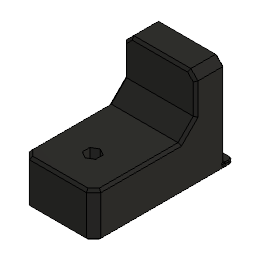
y_idler_bracket (Autodesk Fusion 360 design; units mm, degrees)
Autodesk Fusion 360 part; units mm, degrees
note: some values were not read from the file. Chosen so that the rebuilt part matches the saved one: which face or edge a step refers to; a direction; which pieces of a blend or face edit are solid. Set by a fixed rule: which sketch regions a step uses.
sketch "Sketch1" plane through (0, 0, 0) normal (0, 0, 1) x (1, 0, 0)
  line L0 (0, 13) -> (0, -13) construction
  circle A0 centre (0, 13) radius 1.7
  circle A1 centre (0, -13) radius 1.7
  line L1 (-15, 14.35) -> (15, 14.35)
  line L2 (15, 14.35) -> (15, -21.5)
  line L3 (15, -21.5) -> (-15, -21.5)
  line L4 (-15, -21.5) -> (-15, 14.35)
  line L5 (-15, 19.35) -> (15, 19.35)
  line L6 (15, 19.35) -> (15, 14.35)
  line L7 (-15, 14.35) -> (-15, 19.35)
  line L8 (-15, -18.5) -> (-12, -21.5)
  line L9 (15, -18.5) -> (12, -21.5)
  line L10 (15, 17) -> (-15, 17)
  line L11 (-0.7632, 11.3) -> (0.7632, 11.3)
  line L12 (-1.2042, 11.8) -> (1.2042, 11.8)
  line L13 (1.2704, 11.8704) -> (0.7632, 11.3)
  line L14 (-1.2704, 11.8704) -> (-0.7632, 11.3)
  line L15 (-0.7042, -14.7) -> (0.7042, -14.7)
  line L16 (1.2021, -14.2021) -> (0.7042, -14.7)
  line L17 (0, -13) -> (1.2021, -14.2021) construction
  line L18 (0, -13) -> (-1.2021, -14.2021) construction
  line L19 (-1.2021, -14.2021) -> (-0.7042, -14.7)
  circle A2 centre (0, -13) radius 2.25
  line L20 (-1.591, -14.591) -> (-0.932, -15.25)
  line L21 (1.591, -14.591) -> (0.932, -15.25)
  line L22 (0.932, -15.25) -> (-0.932, -15.25)
  line L23 (-1.4142, -14.75) -> (1.4142, -14.75)
  line L24 (-1.2042, -14.2) -> (1.2042, -14.2) construction
  circle A3 centre (0, 13) radius 2.25
  line L25 (1.0102, 10.75) -> (-1.0102, 10.75)
  line L26 (-1.6814, 11.5049) -> (-1.0102, 10.75)
  line L27 (1.6814, 11.5049) -> (1.0102, 10.75)
  point P0 (0, -13)
  point P1 (0, 13)
  point P2 (0, -15.25)
  point P3 (0, 10.75)
  dimension "d1" = 26
  dimension "d2" = 3.4
  dimension "d3" = 3.4
  dimension "d4" = 30
  dimension "d6" = 8.5
  dimension "d7" = 15
  dimension "d8" = 5
  dimension "d10" = 45
  dimension "d11" = 3
  dimension "d38" = 40.85
  dimension "d60" = 2.35
  dimension "d74" = 0.5
  dimension "d81" = 4.5
  dimension "d82" = 0.5
  dimension "d83" = 0.5
  dimension "d84" = 135
  dimension "d90" = 4.5
  constraint vertical L0
  constraint coincident L0.start A0.centre
  constraint midpoint origin L0
  constraint coincident P0 L0.end
  constraint horizontal L1
  constraint vertical L2
  constraint horizontal L3
  constraint vertical L4
  constraint horizontal L5
  constraint vertical L6
  constraint vertical L7
  constraint coincident L1.start L4.end
  constraint coincident L1.end L2.start
  constraint coincident L4 L8.start
  constraint coincident L3 L8.end
  constraint symmetric L0 L8.start L9.start
  constraint symmetric L0 L8.end L9.end
  constraint coincident P1 L0.start
  constraint coincident L6 L10.start
  constraint coincident L7 L10.end
  constraint horizontal L10
  constraint horizontal L11
  constraint tangent A0 L11
  constraint coincident A0 L12.start
  constraint coincident A0 L12.end
  constraint horizontal L12
  constraint coincident A0 L13.start
  constraint tangent A0 L13
  constraint coincident L11.end L13.end
  constraint coincident A0 L14.start
  constraint tangent A0 L14
  constraint coincident L11.start L14.end
  constraint horizontal L15
  constraint tangent A1 L15
  constraint coincident A1 L16.start
  constraint tangent A1 L16
  constraint coincident L15.end L16.end
  constraint perpendicular L16 L17
  constraint coincident L16.start L17.end
  constraint perpendicular L17 L18
  constraint coincident A1 L18.end
  constraint tangent A1 L19
  constraint coincident L15.start L19.end
  constraint perpendicular L18 L19
  constraint coincident A2 L20.start
  constraint tangent A2 L20
  constraint coincident A2 L21.start
  constraint tangent A2 L21
  constraint horizontal L22
  constraint coincident L20.end L22.end
  constraint tangent A2 L22
  constraint coincident A2 L23.start
  constraint coincident A2 L23.end
  constraint horizontal L23
  constraint coincident A1 L24.start
  constraint coincident A1 L24.end
  constraint horizontal L24
  constraint coincident A2 P2
  constraint coincident L0 P2
  constraint midpoint L22 P2
  constraint parallel L19 L20
  constraint concentric A0 A3
  constraint horizontal L25
  constraint coincident A3 P3
  constraint coincident L0 P3
  constraint midpoint L25 P3
  constraint coincident A3 L26.start
  constraint tangent A3 L26
  constraint coincident A3 L27.start
  constraint tangent A3 L27
  constraint coincident L25.start L27.end
  constraint coincident L25.end L26.end
  constraint parallel L14 L26
  constraint parallel L13 L27
  measures "d1" distance of L0.start P0
  measures "d2" diameter of A0
  measures "d3" diameter of A1
  measures "d4" distance of L1.start L1.end
  measures "d6" distance of P0 L3
  measures "d7" distance of P0 L2
  measures "d8" distance of L5.end L1.end
  measures "d10" angle of L3 L8
  measures "d11" distance of L3.end L8.end
  measures "d38" distance of L3.end L5.start
  measures "d60" distance of L5.end L10.start
  measures "d74" distance of L11 L12
  measures "d81" diameter of A2
  measures "d82" distance of L22 L23
  measures "d83" distance of L15 L24
  measures "d84" angle of L0 L17
  measures "d90" diameter of A3
extrude "Extrude1" add sketch "Sketch1" along normal blind 11.8 contours A0 L1 L12 | A0 L1 L11 L13 L14 A3 | A0 L11 L14 | A0 L12 | A0 L1 A3 | A0 L1 | A0 L11 L13 | L1 L2 L3 L4 L8 L9 A3 L25 L26 L27 | L1 L6 L7 L10 A3 | A3 L25 L26 | L5 L6 L7 L10 | A3 L25 L27 | A1 | A1 L15 L19 | A1 L15 L16 | A2 L23 | A2 L20 L22 | A2 L21 L22 | A2 L23
extrude "Extrude2" add sketch "Sketch1" along normal blind 54.6 contours A0 L1 A3 | A0 L1 | L1 L6 L7 L10 A3 | L5 L6 L7 L10
sketch "Sketch2" plane through (0, 14.35, 0) normal (0, -1, 0) x (1, 0, 0)
  line L0 (-15, 11.8) -> (15, 11.8)
  line L1 (15, 11.8) -> (15, 54.6)
  line L2 (15, 54.6) -> (-15, 54.6)
  line L3 (-15, 54.6) -> (-15, 11.8)
  circle A0 centre (0, 40) radius 1.6
  circle A1 centre (0, 40) radius 2.25
  dimension "d16" = 30
  dimension "d17" = 42.8
  dimension "d18" = 3.2
  dimension "d19" = 15
  dimension "d20" = 14.6
  dimension "d76" = 4.5
  constraint concentric A0 A1
  measures "d16" distance of L1.end L2.end
  measures "d17" distance of L0.end L1.end
  measures "d18" diameter of A0
  measures "d19" horizontal distance of L1.end A0.centre
  measures "d20" vertical distance of L1.end A0.centre
  measures "d76" diameter of A1
extrude "Extrude3" cut sketch "Sketch2" against normal blind 13 contours A0
extrude "Extrude6" cut sketch "Sketch1" along normal blind 6.8 contours A0 L1 L12 | A0 L11 L14 | A0 L12 | A0 L1 | A0 L11 L13 | A1 | A1 L15 L19 | A1 L15 L16
extrude "Extrude9" add sketch "Sketch1" against normal blind 4.2 contours L5 L6 L7 L10
extrude "Extrude11" cut sketch "Sketch2" against normal blind 5 contours A0 | A1
chamfer "Chamfer16" distance 0.625 angle 45 1 edges at (-2.0977, 19.35, 39.1864)
sketch "Sketch5" plane through (-15, 0, 0) normal (-1, 0, 0) x (0, -1, 0)
  line L0 (-17, 0) -> (18.5, 0)
  line L1 (18.5, 0) -> (18.5, 11.8)
  line L2 (18.5, 11.8) -> (-14.35, 11.8)
  line L3 (-14.35, 11.8) -> (-14.35, 54.6)
  line L4 (-14.35, 54.6) -> (-19.35, 54.6)
  line L5 (-19.35, 54.6) -> (-19.35, -4.2)
  line L6 (-19.35, -4.2) -> (-17, -4.2)
  line L7 (-17, -4.2) -> (-17, 0)
  circle A0 centre (-17, 0) radius 0.5
  dimension "d63" = 1
  constraint coincident L0.start L7.end
  measures "d63" diameter of A0
extrude "Extrude10" cut sketch "Sketch5" against normal blind 30 contours L0 L7 A0 | L0 L7 A0
chamfer "Chamfer1" distance 3 angle 45 2 edges at (15, 16.85, 54.6) (-15, 16.85, 54.6)
chamfer "Chamfer11" distance 20 angle 45 1 edges at (0, 14.35, 11.8)
chamfer "Chamfer2" distance 1 angle 45 12 edges at (-15, 14.35, 41.7) (-13.5, 14.35, 53.1) (0, 14.35, 54.6) (13.5, 14.35, 53.1) (15, 14.35, 41.7) (15, -12.075, 11.8) (13.5, -20, 11.8) (0, -21.5, 11.8) (-13.5, -20, 11.8) (-15, -12.075, 11.8) (-15, 4.35, 21.8) (15, 4.35, 21.8)
fillet "Fillet2" radius 2 2 edges at (-15, 18.175, -4.2) (15, 18.175, -4.2)
fillet "Fillet3" radius 0.5 2 edges at (0, 17, -0.5) (0, 16.5, 0)
chamfer "Chamfer14" distance 0.4 angle 45 16 edges at (15, -1.183, 0) (15, 16.384, 0.067) (15, 17.3536, 0.3536) (15, 17.067, -0.616) (15, 17, -1.533) (14.4142, 17, -3.6142) (0, 17, -4.2) (-14.4142, 17, -3.6142) (-15, 17, -1.533) (-15, 17.067, -0.616) (-15, 17.3536, 0.3536) (-15, 16.384, 0.067) (-15, -1.183, 0) (13.5, -20, 0) (0, -21.5, 0) (-13.5, -20, 0)
chamfer "Chamfer15" distance 1 angle 45 8 edges at (-15, 19.35, 24.7) (-14.4142, 19.35, -3.6142) (0, 19.35, -4.2) (14.4142, 19.35, -3.6142) (15, 19.35, 24.7) (-13.5, 19.35, 53.1) (0, 19.35, 54.6) (13.5, 19.35, 53.1)
chamfer "Chamfer17" distance 0.4 angle 45 1 edges at (-2.0977, 14.35, 40.8136)
extrude "Extrude13" cut sketch "Sketch1" along normal blind 5 contours A0 L1 L11 L13 L14 A3 | A0 L11 L14 | A0 L12 | A0 L1 A3 | A0 L11 L13 | A3 L25 L26 | A3 L25 L27 | A1 | A1 L15 L19 | A1 L15 L16 | A2 L23 | A2 L20 L22 | A2 L21 L22 | A2 L23
chamfer "Chamfer20" distance 0.525 angle 45 8 edges at (1.0168, 11.5852, 5) (0, 14.7, 5) (-1.0168, 11.5852, 5) (0, 11.3, 5) (0, -11.3, 5) (0.9531, -14.451, 5) (-0.9531, -14.451, 5) (0, -14.7, 5)
chamfer "Chamfer21" distance 0.4 angle 45 6 edges at (1.3458, 11.1274, 0) (0, 15.25, 0) (-1.3458, 11.1274, 0) (0, -10.75, 0) (-1.2615, -14.9205, 0) (1.2615, -14.9205, 0)
move_body "Move1" bodies 1 to x (-1, 0, 0) y (0, 0, -1) z (0, -1, 0) at (-30, -21.5, -21.5)
move_body "Move2" bodies 1 to x (1, 0, 0) y (0, 1, 0) z (0, 0, 1) at (30, 46.7, 40.85)
delete_face "DeleteFace1" 1 faces at (14.6667, -13.0619, 4.3333)
delete_face "DeleteFace2" 1 faces at (13.8619, -26.5953, 4.6667)
delete_face "DeleteFace3" 1 faces at (4.4714, -28.7333, 4.6667)
delete_face "DeleteFace4" 1 faces at (-12.1953, -28.2619, 4.6667)
delete_face "DeleteFace5" 1 faces at (14.3333, 0.5381, 11.6667)
delete_face "DeleteFace6" 1 faces at (-14.3333, 0.5381, 11.6667)
delete_face "DeleteFace7" 1 faces at (-14.3333, -13.8667, 4.6667)
extrude "Extrude14" add 1 faces at (-0.066, -25.4142, 5) along direction (0, 0, 1) blind 10
delete_face "DeleteFace8" 1 faces at (-1.9548, -16.6138, 0.2083)
sketch "Sketch6" plane through (0, 0, 0) normal (0, 0, -1) x (1, 0, 0)
  line L0 (11.5858, 28.4) -> (-11.5858, 28.4)
  line L1 (-11.5858, 28.4) -> (-14, 25.9858)
  line L2 (-14, 25.9858) -> (-14, -27.4)
  arc A0 (-14, -27.4) -> (-13, -28.4) centre (-13, -27.4) ccw
  line L3 (-13, -28.4) -> (13, -28.4)
  arc A1 (13, -28.4) -> (14, -27.4) centre (13, -27.4) ccw
  line L4 (14, -27.4) -> (14, 25.9858)
  line L5 (14, 25.9858) -> (11.5858, 28.4)
  circle A2 centre (0, 14.8) radius 2.25
  circle A3 centre (0, 14.8) radius 3.5
  circle A4 centre (0, 14.8) radius 1.6
  dimension "d98" = 7
  dimension "d99" = 3.2
  constraint concentric A2 A3
  constraint concentric A3 A4
  measures "d98" diameter of A3
  measures "d99" diameter of A4
extrude "Extrude15" add sketch "Sketch6" against normal up to surface (15 mm away) contours A2 | A3
extrude "Extrude16" add 1 faces at (-0.0399, -25.0652, 15) along direction (0, 0, 1) blind 3.6
sketch "Sketch7" plane through (15, 0, 0) normal (1, 0, 0) x (0, 1, 0)
  line L0 (14.4, 26) -> (-6.6, 5)
  line L1 (-6.6, 5) -> (-6.6, 18.6)
  line L2 (-6.6, 18.6) -> (-26.4, 18.6)
  line L3 (-26.4, 18.6) -> (-26.4, 1)
  line L4 (-26.4, 1) -> (27.4, 1)
  line L5 (27.4, 1) -> (27.4, 1.95)
  line L6 (27.4, 1.95) -> (26.066, 1.95)
  arc A0 (26.066, 1.95) -> (25.9794, 1.9) centre (26.066, 1.85) ccw
  arc A1 (24.75, 3.1294) -> (25.9794, 1.9) centre (25.2, 2.35) ccw
  arc A2 (24.75, 3.1294) -> (24.8, 3.216) centre (24.7, 3.216) ccw
  line L7 (24.8, 3.216) -> (24.8, 37.85)
  line L8 (24.8, 37.85) -> (14.4, 37.85)
  line L9 (14.4, 37.85) -> (14.4, 26)
  line L10 (-6.6, 18.6) -> (7, 18.6)
  constraint coincident L1.end L2.start
  constraint coincident L0 L10.end
  constraint perpendicular L1 L10
extrude "Extrude17" add sketch "Sketch7" against normal up to surface (30 mm away) contours L0 L1 L10
sketch "Sketch8" plane through (0, 0, 18.6) normal (0, 0, 1) x (-1, 0, 0)
  circle A0 centre (0, 14.8) radius 1.6
  line L0 (15, 26.4) -> (12, 29.4)
  line L1 (12, 29.4) -> (-12, 29.4)
  line L2 (-12, 29.4) -> (-15, 26.4)
  line L3 (-15, 26.4) -> (-15, -7)
  line L4 (-15, -7) -> (15, -7)
  line L5 (15, -7) -> (15, 26.4)
  circle A1 centre (0, 14.8) radius 1.55
  line L6 (2.75, 16.3877) -> (0, 17.9754)
  line L7 (0, 17.9754) -> (-2.75, 16.3877)
  line L8 (-2.75, 16.3877) -> (-2.75, 13.2123)
  line L9 (-2.75, 13.2123) -> (0, 11.6246)
  line L10 (0, 11.6246) -> (2.75, 13.2123)
  line L11 (2.75, 13.2123) -> (2.75, 16.3877)
  circle A2 centre (0, 14.8) radius 1.6
  line L12 (15, 26.4) -> (12, 29.4)
  line L13 (12, 29.4) -> (-12, 29.4)
  line L14 (-12, 29.4) -> (-15, 26.4)
  line L15 (-15, 26.4) -> (-15, -7)
  line L16 (-15, -7) -> (15, -7)
  line L17 (15, -7) -> (15, 26.4)
  point P0 (0, 14.8)
  dimension "d107" = 2.75
  constraint coincident P0 A0.centre
  measures "d107" distance of P0 L11
extrude "Extrude18" cut sketch "Sketch8" against normal blind 5 contours L6 L7 L8 L9 L10 L11
chamfer "Chamfer23" distance 1 angle 45 7 edges at (15, 10.7, 22.3) (15, -9.7, 18.6) (13.5, -27.9, 18.6) (0, -29.4, 18.6) (-13.5, -27.9, 18.6) (-15, -9.7, 18.6) (-15, 10.7, 22.3)
sketch "Sketch10" plane through (0, 0, 0) normal (0, 0, -1) x (1, 0, 0)
  circle A0 centre (0, 14.8) radius 1.6
  line L0 (11.5858, 28.4) -> (-11.5858, 28.4)
  line L1 (-11.5858, 28.4) -> (-14, 25.9858)
  line L2 (-14, 25.9858) -> (-14, -27.4)
  arc A1 (-14, -27.4) -> (-13, -28.4) centre (-13, -27.4) ccw
  line L3 (-13, -28.4) -> (13, -28.4)
  arc A2 (13, -28.4) -> (14, -27.4) centre (13, -27.4) ccw
  line L4 (14, -27.4) -> (14, 25.9858)
  line L5 (14, 25.9858) -> (11.5858, 28.4)
  circle A3 centre (0, 14.8) radius 3.1
  dimension "d117" = 6.2
  constraint concentric A0 A3
  measures "d117" diameter of A3
extrude "Extrude20" cut sketch "Sketch10" against normal blind 3 contours A3
chamfer "Chamfer27" distance 0.2 angle 45 1 edges at (-2.8902, -15.921, 0)
chamfer "Chamfer28" distance 0.2 angle 45 1 edges at (-1.4917, -14.2214, 3)
sketch "Sketch11" plane through (0, 0, 3) normal (0, 0, -1) x (1, 0, 0)
  circle A0 centre (0, 14.8) radius 3.1
  circle A1 centre (0, 14.8) radius 1.8 construction
  line L0 (0, 14.8) -> (1, 14.8) construction
  line L1 (-2.5232, 12.999) -> (2.5232, 12.999)
  line L2 (-2.5232, 16.601) -> (2.5232, 16.601)
  line L3 (0, 14.8) -> (0, 12.999) construction
  line L4 (0, 14.8) -> (0, 16.601) construction
  dimension "d122" = 1.801
  dimension "d123" = 1.801
  constraint coincident A0.centre A1.centre
  constraint parallel L0 L1
  constraint parallel L0 L2
  constraint perpendicular L1 L3
  constraint coincident L1 L3.end
  constraint perpendicular L2 L4
  constraint coincident L2 L4.end
  constraint coincident A0 L1.start
  constraint coincident A0 L1.end
  constraint coincident A0 L2.start
  constraint coincident A0 L2.end
  measures "d122" distance of A0.centre L3.end
  measures "d123" distance of A0.centre L4.end
extrude "Extrude21" cut sketch "Sketch11" against normal blind 0.2 contours A0 L1 L2
sketch "Sketch12" plane through (0, 0, 3.2) normal (0, 0, -1) x (1, 0, 0)
  circle A0 centre (0, 14.8) radius 1.6 construction
  line L0 (-2.5232, 12.999) -> (2.5232, 12.999)
  arc A1 (2.5232, 12.999) -> (2.5232, 16.601) centre (0, 14.8) ccw
  line L1 (2.5232, 16.601) -> (-2.5232, 16.601)
  arc A2 (-2.5232, 16.601) -> (-2.5232, 12.999) centre (0, 14.8) ccw
  line L2 (0, 14.8) -> (1, 14.8) construction
  line L3 (0, 14.8) -> (0, 15.8) construction
  line L4 (1.601, 12.999) -> (1.601, 16.601)
  line L5 (-1.601, 12.999) -> (-1.601, 16.601)
  line L6 (0, 14.8) -> (1.601, 14.8) construction
  line L7 (0, 14.8) -> (-1.601, 14.8) construction
  dimension "d126" = 90
  dimension "d127" = 1.601
  dimension "d128" = 1.601
  constraint coincident A0.centre A1.centre
  constraint parallel L3 L4
  constraint parallel L3 L5
  constraint perpendicular L4 L6
  constraint coincident L4 L6.end
  constraint perpendicular L5 L7
  constraint coincident L5 L7.end
  constraint coincident L0 L4.start
  constraint coincident L1 L4.end
  constraint coincident L0 L5.start
  constraint coincident L1 L5.end
  measures "d126" angle of L2 L3
  measures "d127" distance of A0.centre L6.end
  measures "d128" distance of A0.centre L7.end
extrude "Extrude22" cut sketch "Sketch12" against normal blind 0.2 contours L0 L1 L4 L5
extrude "Extrude23" add 1 faces at (-1.2572, -13.4199, 3.4) along direction (0, 0, -1) up to surface (0.2 mm away)
extrude "Extrude24" add 3 faces at (2.1007, -14.8, 3.2) (-2.0982, -14.7289, 3.2) (-1.2572, -13.4199, 3.2) along direction (0, 0, -1) up to surface end surface through (0, 0, 3) normal (0, 0, -1) offset 0
delete_face "DeleteFace17" 1 faces at (3.2173, -14.4781, 0.0667)
sketch "Sketch13" plane through (0, 0, 0) normal (0, 0, -1) x (1, 0, 0)
  line L0 (11.5858, 28.4) -> (-11.5858, 28.4)
  line L1 (-11.5858, 28.4) -> (-14, 25.9858)
  line L2 (-14, 25.9858) -> (-14, -27.4)
  arc A0 (-14, -27.4) -> (-13, -28.4) centre (-13, -27.4) ccw
  line L3 (-13, -28.4) -> (13, -28.4)
  arc A1 (13, -28.4) -> (14, -27.4) centre (13, -27.4) ccw
  line L4 (14, -27.4) -> (14, 25.9858)
  line L5 (14, 25.9858) -> (11.5858, 28.4)
  circle A2 centre (0, 14.8) radius 3.1
  line L6 (-2.75, 13.2123) -> (0, 11.6246)
  line L7 (0, 11.6246) -> (2.75, 13.2123)
  line L8 (2.75, 13.2123) -> (2.75, 16.3877)
  line L9 (2.75, 16.3877) -> (0, 17.9754)
  line L10 (0, 17.9754) -> (-2.75, 16.3877)
  line L11 (-2.75, 16.3877) -> (-2.75, 13.2123)
  point P0 (0, 14.8)
  dimension "d135" = 2.75
  constraint coincident P0 A2.centre
  measures "d135" distance of P0 L11
move_face "OffsetFaces1" offset 1.3 1 faces at (3.0846, -14.4913, 1)
extrude "Extrude25" cut sketch "Sketch13" against normal blind 2.4 contours A2 L6 L7 L8 L9 L10 L11
chamfer "Chamfer29" distance 0.4 angle 45 12 edges at (1.375, -12.4184, 0) (0, -11.7, 0) (-1.375, -12.4184, 0) (-2.6847, -13.25, 0) (-2.75, -14.8, 0) (-2.6847, -16.35, 0) (-1.375, -17.1816, 0) (0, -17.9, 0) (1.375, -17.1816, 0) (2.6847, -16.35, 0) (2.75, -14.8, 0) (2.6847, -13.25, 0)
extrude "Extrude26" add 1 faces at (1.1833, -16.8496, 13.6) along direction (0, 0, 1) blind 1
sketch "Sketch14" plane through (0, 0, 2.4) normal (0, 0, -1) x (1, 0, 0)
  circle A0 centre (0, 14.8) radius 1.8 construction
  arc A1 (-2.6142, 16.4661) -> (-2.75, 16.2309) centre (0, 14.8) ccw
  line L0 (-2.75, 16.2309) -> (-2.75, 13.3691)
  arc A2 (-2.75, 13.3691) -> (-2.6142, 13.1339) centre (0, 14.8) ccw
  line L1 (-2.6142, 13.1339) -> (-0.1358, 11.703)
  arc A3 (-0.1358, 11.703) -> (0.1358, 11.703) centre (0, 14.8) ccw
  line L2 (0.1358, 11.703) -> (2.6142, 13.1339)
  arc A4 (2.6142, 13.1339) -> (2.75, 13.3691) centre (0, 14.8) ccw
  line L3 (2.75, 13.3691) -> (2.75, 16.2309)
  arc A5 (2.75, 16.2309) -> (2.6142, 16.4661) centre (0, 14.8) ccw
  line L4 (2.6142, 16.4661) -> (0.1358, 17.897)
  arc A6 (0.1358, 17.897) -> (-0.1358, 17.897) centre (0, 14.8) ccw
  line L5 (-0.1358, 17.897) -> (-2.6142, 16.4661)
  line L6 (0, 14.8) -> (1, 14.8) construction
  line L7 (-2.3806, 12.999) -> (2.3806, 12.999)
  line L8 (-2.3806, 16.601) -> (2.3806, 16.601)
  line L9 (0, 14.8) -> (0, 12.999) construction
  line L10 (0, 14.8) -> (0, 16.601) construction
  dimension "d142" = 1.801
  dimension "d143" = 1.801
  constraint coincident A0.centre A1.centre
  constraint parallel L6 L7
  constraint parallel L6 L8
  constraint perpendicular L7 L9
  constraint coincident L7 L9.end
  constraint perpendicular L8 L10
  constraint coincident L8 L10.end
  constraint coincident L1 L7.start
  constraint coincident L2 L7.end
  constraint coincident L5 L8.start
  constraint coincident L4 L8.end
  measures "d142" distance of A0.centre L9.end
  measures "d143" distance of A0.centre L10.end
extrude "Extrude27" cut sketch "Sketch14" against normal blind 0.2 contours A1 L0 A2 L1 L2 A4 L3 A5 L4 L5 L7 L8
sketch "Sketch15" plane through (0, 0, 2.6) normal (0, 0, -1) x (1, 0, 0)
  circle A0 centre (0, 14.8) radius 1.8 construction
  arc A1 (-2.6142, 16.4661) -> (-2.75, 16.2309) centre (0, 14.8) ccw
  line L0 (-2.75, 16.2309) -> (-2.75, 13.3691)
  arc A2 (-2.75, 13.3691) -> (-2.6142, 13.1339) centre (0, 14.8) ccw
  line L1 (-2.6142, 13.1339) -> (-2.3806, 12.999)
  line L2 (-2.3806, 12.999) -> (2.3806, 12.999)
  line L3 (2.3806, 12.999) -> (2.6142, 13.1339)
  arc A3 (2.6142, 13.1339) -> (2.75, 13.3691) centre (0, 14.8) ccw
  line L4 (2.75, 13.3691) -> (2.75, 16.2309)
  arc A4 (2.75, 16.2309) -> (2.6142, 16.4661) centre (0, 14.8) ccw
  line L5 (2.6142, 16.4661) -> (2.3806, 16.601)
  line L6 (2.3806, 16.601) -> (-2.3806, 16.601)
  line L7 (-2.3806, 16.601) -> (-2.6142, 16.4661)
  line L8 (0, 14.8) -> (1, 14.8) construction
  line L9 (0, 14.8) -> (0, 15.8) construction
  line L10 (1.801, 12.999) -> (1.801, 16.601)
  line L11 (-1.801, 12.999) -> (-1.801, 16.601)
  line L12 (0, 14.8) -> (1.801, 14.8) construction
  line L13 (0, 14.8) -> (-1.801, 14.8) construction
  dimension "d146" = 90
  dimension "d147" = 1.801
  dimension "d148" = 1.801
  constraint coincident A0.centre A1.centre
  constraint parallel L9 L10
  constraint parallel L9 L11
  constraint perpendicular L10 L12
  constraint coincident L10 L12.end
  constraint perpendicular L11 L13
  constraint coincident L11 L13.end
  constraint coincident L2 L10.start
  constraint coincident L6 L10.end
  constraint coincident L2 L11.start
  constraint coincident L6 L11.end
  measures "d146" angle of L8 L9
  measures "d147" distance of A0.centre L12.end
  measures "d148" distance of A0.centre L13.end
extrude "Extrude28" cut sketch "Sketch15" against normal blind 0.2 contours L2 L6 L10 L11
equation "d3 = d2"
equation "d7 = d4 / 2"
equation "d14 = 38 mm + 10 mm + 6.6 mm"
equation "d19 = d16 / 2"
equation "d20 = 8 mm + 6.6 mm"
equation "d38 = 38.5 mm + 2.35 mm"
equation "d42 = 11 mm - 4.2 mm"
equation "d107 = ( 5.5 / 2 ) * 1 mm"
